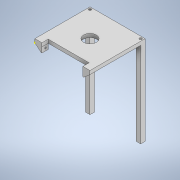
# Autodesk Inventor part: Haltung_Presse
Saved by Autodesk Inventor 2020.3 (Build 243373000, 373)
## iProperties
Created: 2021-10-01
Part Number: Haltung_Presse
Material: Generisch
Document SubType Name: Modeling
Designer: Preuß P. Ch.
Density: 1 g/cm^3
Appearance: Vorgabe
Author: Preuß P. Ch.
Autodesk Inventor part; units mm, degrees
ref_plane "YZ Plane" through (0, 0, 0) normal (1, 0, 0) x (0, 1, 0)
ref_plane "XZ Plane" through (0, 0, 0) normal (0, 1, 0) x (-1, 0, 0)
ref_plane "XY Plane" through (0, 0, 0) normal (0, 0, 1) x (1, 0, 0)
sketch "Skizze5" plane through (0, 0, 0) normal (0, 1, 0) x (-1, 0, 0)
  line L0 (0, 0) -> (-310, 0)
  line L1 (-310, 0) -> (-310, -310)
  line L2 (-310, -310) -> (0, -310)
  line L3 (0, -310) -> (0, 0)
  dimension "d14" = 310
  dimension "d15" = 310
  constraints: 8 end point, 2 parallel, 1 horizontal, 1 perpendicular
  measures "d14" distance of L2.end L1.end
  measures "d15" distance of L1.end L0.end
extrude "Extrusion5" add sketch "Skizze5" along normal blind 500
sketch "Skizze6" plane through (0, 500, 0) normal (0, 1, 0) x (1, 0, 0)
  line L0 (0, 310) -> (0, 0) projected
  line L1 (0, 0) -> (310, 0) projected
  line L2 (40, 35) -> (270, 35)
  line L3 (270, 35) -> (270, 0)
  line L4 (270, 0) -> (40, 0)
  line L5 (40, 0) -> (40, 35)
  dimension "d20" = 230
  constraints: 8 end point, 2 parallel, 1 horizontal, 1 perpendicular, 1 point on line
  measures "d20" distance of L3.end L4.end
extrude "Extrusion6" cut sketch "Skizze6" against normal blind 500
sketch "Skizze7" plane through (0, 0, 0) normal (0, -1, 0) x (1, 0, 0)
  line L0 (310, 0) -> (310, -310) projected
  line L1 (40, -35) -> (270, -35) projected
  line L2 (310, 0) -> (270, 0)
  line L3 (270, 0) -> (270, -35)
  line L4 (270, -35) -> (310, -35)
  line L5 (310, -35) -> (310, 0)
  line L6 (40, 0) -> (40, -35) projected
  line L7 (0, -310) -> (0, 0) projected
  line L8 (40, 0) -> (0, 0)
  line L9 (0, 0) -> (0, -35)
  line L10 (0, -35) -> (40, -35)
  line L11 (40, -35) -> (40, 0)
  line L12 (310, -35) -> (0, -35)
  line L13 (0, -35) -> (0, -285)
  line L14 (0, -285) -> (310, -285)
  line L15 (310, -285) -> (310, -35)
  line L16 (310, -310) -> (0, -310) projected
  line L17 (310, -285) -> (285, -285)
  line L18 (285, -285) -> (285, -310)
  line L19 (285, -310) -> (310, -310)
  line L20 (310, -310) -> (310, -285)
  line L21 (0, -285) -> (25, -285)
  line L22 (25, -285) -> (25, -310)
  line L23 (25, -310) -> (0, -310)
  line L24 (0, -310) -> (0, -285)
  dimension "d23" = 250
  dimension "d24" = 25
  dimension "d25" = 25
  constraints: 40 end point, 10 parallel, 5 horizontal, 5 perpendicular, 5 point on line
  measures "d23" distance of L13.end L12.end
  measures "d24" distance of L19.end L18.end
  measures "d25" distance of L22.end L23.end
extrude "Extrusion7" cut sketch "Skizze7" against normal blind 480 contours L0 L4 L3 L2 | L0 L14 L7 L10 L1 L4 | L18 L16 L22 L14 | L10 L7 L8 L6
sketch "Skizze8" plane through (0, 500, 0) normal (0, 1, 0) x (1, 0, 0)
  line L0 (0, 0) -> (40, 0) projected
  circle A0 centre (155, 155) radius 36
  dimension "d30" = 72
  constraints: 1 centre point
  measures "d30" diameter of A0
extrude "Extrusion8" cut sketch "Skizze8" against normal blind 20
sketch "Skizze9" plane through (0, 480, 0) normal (0, -1, 0) x (1, 0, 0)
  point P0 (0, 0)
sketch "Skizze10" plane through (0, 480, 0) normal (0, -1, 0) x (1, 0, 0)
  line L0 (270, 0) -> (310, 0) projected
  line L1 (270, 0) -> (275, 0)
  line L2 (275, 0) -> (275, -35)
  line L3 (275, -35) -> (270, -35)
  line L4 (270, -35) -> (270, 0)
  line L5 (39.9329, 0) -> (34.9329, 0)
  line L6 (34.9329, 0) -> (34.9329, -35)
  line L7 (34.9329, -35) -> (39.9329, -35)
  line L8 (39.9329, -35) -> (39.9329, 0)
  point P0 (0, 0)
  dimension "d33" = 5
  dimension "d34" = 35
  dimension "d35" = 5
  constraints: 16 end point, 4 parallel, 2 horizontal, 2 perpendicular, 2 point on line
  measures "d33" distance of L2.end L3.end
  measures "d34" distance of L1.end L2.end
  measures "d35" distance of L7.end L6.end
extrude "Extrusion9" add sketch "Skizze10" along normal blind 30
sketch "Skizze11" plane through (0, 500, 0) normal (0, 0, 1) x (1, 0, 0)
  line L0 (0, -20) -> (0, 0) projected
  line L1 (0, -20) -> (34.9329, -20) projected
  line L2 (0, -20) -> (34.9329, -20)
  line L3 (39.9329, -50) -> (34.9329, -50) projected
  line L4 (34.9329, -20) -> (34.9329, -50)
  line L5 (34.9329, -50) -> (0, -20)
  line L6 (275, -20) -> (310, -20) projected
  line L7 (310, -20) -> (275, -20)
  line L8 (275, -20) -> (275, -50) projected
  line L9 (275, -20) -> (275, -50)
  line L10 (275, -50) -> (310, -20)
  point P0 (0, -500)
  constraints: 12 end point, 2 perpendicular, 1 collinear, 1 horizontal
extrude "Extrusion10" add sketch "Skizze11" against normal blind 5
sketch "Skizze12" plane through (34.9329, 450, -35) normal (-1, 0, 0) x (0, 0, 1)
  line L0 (30, 0) -> (0, 0) projected
  line L1 (0, 0) -> (15, 0)
  line L2 (15, 0) -> (15, 15)
  line L3 (15, 15) -> (0, 15)
  line L4 (0, 15) -> (0, 0)
  point P0 (35, -450)
  dimension "d40" = 15
  dimension "d41" = 15
  constraints: 8 end point, 2 parallel, 1 horizontal, 1 perpendicular
  measures "d40" distance of L3.end L2.end
  measures "d41" distance of L2.end L1.end
hole "Bohrung1" at (34.9329, 465, -20) direction (1, 0, 0) diameter 10 depth 27.3 tip angle 118
sketch "Skizze13" plane through (275, 450, -35) normal (1, 0, 0) x (0, 0, -1)
  line L0 (0, 0) -> (-15, 0)
  line L1 (-15, 0) -> (-15, 15)
  line L2 (-15, 15) -> (0, 15)
  line L3 (0, 15) -> (0, 0)
  point P0 (-35, -450)
  dimension "d49" = 15
  dimension "d50" = 15
  constraints: 8 end point, 2 parallel, 1 horizontal, 1 perpendicular
  measures "d49" distance of L1.end L2.end
  measures "d50" distance of L0.end L1.end
hole "Bohrung2" at (275, 465, -20) direction (-1, 0, 0) diameter 10 depth 27.3 tip angle 118
chamfer "Fase1" distance 2 angle 45 1 edges at (34.9329, 465, -25)
chamfer "Fase2" distance 2 angle 45 1 edges at (275, 465, -15)
sketch "Skizze14" plane through (0, 500, 0) normal (0, 1, 0) x (1, 0, 0)
  line L0 (310, 0) -> (310, 310) projected
  line L1 (310, 310) -> (297.5, 310)
  line L2 (297.5, 310) -> (297.5, 297.5)
  line L3 (297.5, 297.5) -> (310, 297.5)
  line L4 (310, 297.5) -> (310, 310)
  line L5 (0, 310) -> (0, 285) projected
  line L6 (0, 310) -> (12.5, 310)
  line L7 (12.5, 310) -> (12.5, 297.5)
  line L8 (12.5, 297.5) -> (0, 297.5)
  line L9 (0, 297.5) -> (0, 310)
  point P0 (0, 0)
  dimension "d64" = 12.5
  dimension "d65" = 12.5
  dimension "d66" = 12.5
  dimension "d67" = 12.5
  constraints: 16 end point, 4 parallel, 2 horizontal, 2 perpendicular
  measures "d64" distance of L3.end L2.end
  measures "d65" distance of L2.end L1.end
  measures "d66" distance of L7.end L8.end
  measures "d67" distance of L6.end L7.end
hole "Bohrung3" at (12.5, 500, -297.5) at (297.5, 500, -297.5) direction (0, -1, 0) diameter 10 depth 27.3 tip angle 118
chamfer "Fase3" distance 2 angle 45 2 edges at (297.5, 500, -302.5) (12.5, 500, -302.5)
